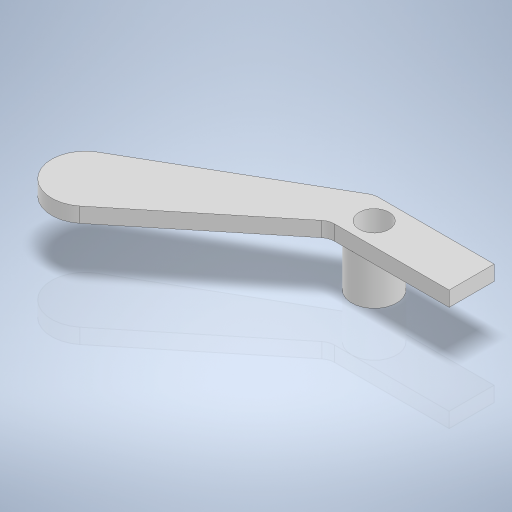
# Autodesk Inventor part: 1 part 12
Saved by Autodesk Inventor 2024 (Build 280153000, 153)
## iProperties
Created: 2024-07-30
Part Number: 1 part 12
Material: Generisch
Document SubType Name: Modeling
Designer: ffogue
Density: 1 g/cm^3
Appearance: Vorgabe
Author: ffogue
Autodesk Inventor part; units mm, degrees
ref_plane "YZ Plane" through (0, 0, 0) normal (1, 0, 0) x (0, 1, 0)
ref_plane "XZ Plane" through (0, 0, 0) normal (0, 1, 0) x (-1, 0, 0)
ref_plane "XY Plane" through (0, 0, 0) normal (0, 0, 1) x (1, 0, 0)
sketch "Skizze1" plane through (0, 0, 0) normal (0, 0, 1) x (1, 0, 0)
  line L0 (0, 0) -> (0, 6)
  line L1 (0, 6) -> (-23.3827, -7.5)
  arc A0 (-23.3827, -7.5) -> (-18.3295, -14.9173) centre (-21.1327, -11.3971) ccw
  line L2 (-18.3295, -14.9173) -> (0, 0)
  line L3 (0, 6) -> (16, 6)
  line L4 (16, 6) -> (16, 0)
  line L5 (16, 0) -> (0, 0)
  line L6 (-21.1327, -11.3971) -> (0, 3) construction
  dimension "d1" = 6
  dimension "d3" = 30
  dimension "d4" = 4.5
  dimension "d5" = 16
  dimension "d6" = 27
  constraints: 14 end point, 2 perpendicular, 2 point on circle, 1 centre point, 1 horizontal, 1 midpoint, 1 symmetric about line, 1 tangent, 1 vertical
  measures "d1" distance of L0.start L0.end
  measures "d3" angle of L1 L3
  measures "d4" radius of A0
  measures "d5" distance between parallel lines of L4 L0
  measures "d6" distance of L1.end L0.end
extrude "Extrusion1" add sketch "Skizze1" along normal mid plane 2
sketch "Skizze2" plane through (0, 0, -1) normal (0, 0, -1) x (-1, 0, 0)
  circle A0 centre (-3, 3) radius 3
  line L0 (-16, 6) -> (-16, 0) projected
  point P0 (0, 0)
  point P1 (-16, 3)
  dimension "d9" = 6
  dimension "d10" = 13
  constraints: 1 centre point, 1 horizontal alignment, 1 midpoint
  measures "d9" diameter of A0
  measures "d10" distance from line of L0 A0.centre
extrude "Extrusion2" add sketch "Skizze2" along normal blind 6
sketch "Skizze3" plane through (3, 3, -7) normal (0, 0, -1) x (-1, 0, 0)
  circle A0 centre (0, 0) radius 3 projected
  point P0 (3, -3)
  constraints: 1 coincident
hole "Bohrung1" at (3, 3, -7) direction (0, 0, 1) diameter 4 depth 8
fillet "Rundung1" radius 2 2 edges at (0, 6, 0) (0, 0, 0)
